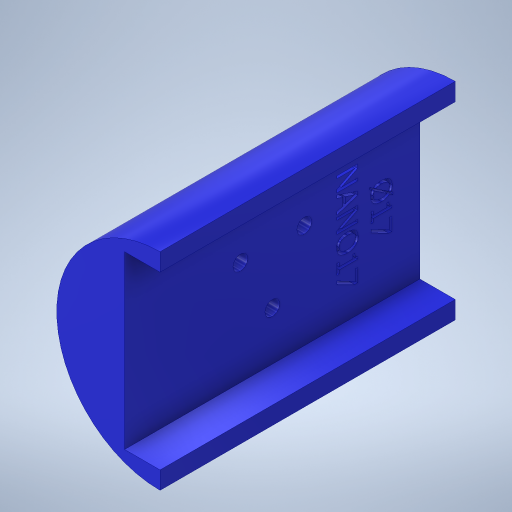
# Autodesk Inventor part: NANO17Shell18_B
Saved by Autodesk Inventor 2023 (Build 270158000, 158)
## iProperties
Created: 2016-07-01
Part Number: NANO17Shell18_B
Material: ABS Plastic
Document SubType Name: Modeling
Designer: Administrateur
Density: 1.06 g/cm^3
Appearance: Blue - Wall Paint - Glossy
Author: Administrateur
Autodesk Inventor part; units mm, degrees
ref_plane "XZ Plane" through (0, 0, 0) normal (0, 1, 0) x (-1, 0, 0)
sketch "Sketch1" plane through (0, 0, 0) normal (0, 0, 1) x (1, 0, 0)
  arc A0 (0, 17.5) -> (0, -17.5) centre (0, 0) ccw
  line L0 (0, 17.5) -> (0, 14.5)
  line L1 (0, 14.5) -> (-6, 14.5)
  line L2 (-6, 14.5) -> (-6, 0)
  line L3 (-46.5484, 0) -> (26.4312, 0) construction
  line L4 (0, -17.5) -> (0, -14.5)
  line L5 (0, -14.5) -> (-6, -14.5)
  line L6 (-6, -14.5) -> (-6, 0)
  dimension "d2" = 17.5
  dimension "d3" = 29
  dimension "d4" = 6
  dimension "d27" = 14.5
  dimension "d28" = 3
  constraints: 14 end point, 2 horizontal, 2 point on circle, 2 symmetric about line, 1 centre point, 1 coincident, 1 perpendicular, 1 vertical
  measures "d2" radius of A0
  measures "d3" distance between parallel lines of L5 L1
  measures "d4" distance of L0.end L1.end
  measures "d27" distance of L1.end L2.end
  measures "d28" distance of L0.start L0.end
extrude "Extrusion1" add sketch "Sketch1" along normal blind 50
sketch "Sketch2" plane through (-6, -14.5, 0) normal (1, 0, 0) x (0, 0, -1)
  line L0 (-25, 14.5) -> (-50, 14.5) construction
  line L1 (-50, 32) -> (-50, -3) construction
  line L2 (0, 32) -> (-50, 32) construction
  line L3 (-25, 32) -> (-25, -3) construction
  line L4 (0, -3) -> (-50, -3) construction
  circle A0 centre (-25, 14.5) radius 6.25 construction
  line L5 (-25, 14.5) -> (-30.4127, 17.625) construction
  line L6 (-25, 14.5) -> (-25, 8.25) construction
  line L7 (-25, 14.5) -> (-19.5873, 17.625) construction
  point P0 (0, 14.5)
  dimension "d6" = 12.5
  dimension "d7" = 30
  dimension "d10" = 360
  constraints: 10 end point, 4 coincident, 4 midpoint, 13 other
  measures "d7" angle of L0 L5
hole "Hole1" at (-6, -6.25, 25) at (-6, 3.125, 19.5873) at (-6, 3.125, 30.4127) direction (-1, 0, 0) diameter 2.5 end through all
ref_plane "Work Plane1" through (-17.5, 0, 0) normal (1, 0, 0) x (0, 1, 0)
sketch "Sketch3" plane through (-17.5, 0, 0) normal (1, 0, 0) x (0, 1, 0)
  line L0 (17.5, 0) -> (-17.5, 0) projected
  line L1 (-17.5, 0) -> (-17.5, 50) projected
  line L2 (17.5, 50) -> (-17.5, 50) projected
  line L3 (17.5, 0) -> (17.5, 50) projected
  circle A0 centre (3.125, 30.4127) radius 1.25 projected
  circle A1 centre (3.125, 19.5873) radius 1.25 projected
  line L4 (3.125, 30.4127) -> (3.125, 19.5873) construction
  circle A2 centre (-6.25, 25) radius 1.25 projected
  line L5 (3.125, 19.5873) -> (-6.25, 25) construction
  line L6 (-6.25, 25) -> (3.125, 30.4127) construction
  point P0 (0, 0)
  point P1 (3.125, 30.4127)
  point P2 (3.125, 19.5873)
  point P3 (-6.25, 25)
  constraints: 6 end point, 3 coincident, 3 horizontal alignment, 3 other
ref_plane "Work Plane2" through (-10, 0, 0) normal (1, 0, 0) x (0, 1, 0)
hole "Hole2" at (-17.5, 3.125, 30.4127) at (-17.5, 3.125, 19.5873) at (-17.5, -6.25, 25) direction (1, 0, 0) diameter 5 depth 7.5
sketch "Esquisse4" plane through (-6, -14.5, 0) normal (1, 0, 0) x (0, 0, -1)
  line L0 (-4.5555, 21.4204) -> (-4.5555, 5.6534) construction
  line L1 (-4.5555, 5.6534) -> (-13.9713, 5.6534) construction
  line L2 (-13.9713, 5.6534) -> (-13.9713, 21.4204) construction
  line L3 (-13.9713, 21.4204) -> (-4.5555, 21.4204) construction
  spline S0 degree 2 poles (-6.521, 14.6161) (-7.3889, 14.6161) (-8.3448, 15.4613) (-8.3448, 16.1647) knots 0 0 0 1 2 2 2
  spline S1 degree 2 poles (-8.3448, 16.1647) (-8.3448, 16.4228) (-8.2086, 16.8681) (-8.0838, 17.0468) knots 0 0 0 1 2 2 2
  line L4 (-8.0838, 17.0468) -> (-8.5433, 17.3588)
  line L5 (-8.5433, 17.3588) -> (-8.5433, 17.7049)
  line L6 (-8.5433, 17.7049) -> (-7.8909, 17.2624)
  spline S2 degree 2 poles (-7.8909, 17.2624) (-7.6584, 17.4723) (-6.972, 17.7105) (-6.521, 17.7105) knots 0 0 0 1 2 2 2
  spline S3 degree 2 poles (-6.521, 17.7105) (-5.6559, 17.7105) (-4.6973, 16.8625) (-4.6973, 16.1647) knots 0 0 0 1 2 2 2
  spline S4 degree 2 poles (-4.6973, 16.1647) (-4.6973, 15.8953) (-4.8277, 15.4755) (-4.9554, 15.2883) knots 0 0 0 1 2 2 2
  line L7 (-4.9554, 15.2883) -> (-4.5555, 15.0189)
  line L8 (-4.5555, 15.0189) -> (-4.5555, 14.67)
  line L9 (-4.5555, 14.67) -> (-5.1454, 15.0728)
  spline S5 degree 2 poles (-5.1454, 15.0728) (-5.378, 14.8572) (-6.053, 14.6161) (-6.521, 14.6161) knots 0 0 0 1 2 2 2
  spline S6 degree 2 poles (-6.521, 15.0955) (-6.1977, 15.0955) (-5.69, 15.2259) (-5.5226, 15.3337) knots 0 0 0 1 2 2 2
  line L10 (-5.5226, 15.3337) -> (-7.7264, 16.8086)
  spline S7 degree 2 poles (-7.7264, 16.8086) (-7.8342, 16.6753) (-7.942, 16.3746) (-7.942, 16.1619) knots 0 0 0 1 2 2 2
  spline S8 degree 2 poles (-7.942, 16.1619) (-7.942, 15.6769) (-7.2102, 15.0955) (-6.521, 15.0955) knots 0 0 0 1 2 2 2
  spline S9 degree 2 poles (-5.3099, 15.5266) (-5.205, 15.6485) (-5.1, 15.969) (-5.1, 16.1619) knots 0 0 0 1 2 2 2
  spline S10 degree 2 poles (-5.1, 16.1619) (-5.1, 16.6498) (-5.8233, 17.2312) (-6.521, 17.2312) knots 0 0 0 1 2 2 2
  spline S11 degree 2 poles (-6.521, 17.2312) (-6.8387, 17.2312) (-7.3322, 17.1092) (-7.508, 16.9986) knots 0 0 0 1 2 2 2
  line L11 (-7.508, 16.9986) -> (-5.3099, 15.5266)
  line L12 (-8.271, 12.2223) -> (-8.271, 13.9297)
  line L13 (-8.271, 13.9297) -> (-7.9136, 13.9297)
  line L14 (-7.9136, 13.9297) -> (-7.9136, 13.2944)
  line L15 (-7.9136, 13.2944) -> (-5.568, 13.2944)
  line L16 (-5.568, 13.2944) -> (-5.568, 13.9297)
  line L17 (-5.568, 13.9297) -> (-5.2475, 13.9297)
  spline S12 degree 2 poles (-5.2475, 13.9297) (-5.2475, 13.5695) (-5.0433, 13.2292) (-4.7597, 13.2065) knots 0 0 0 1 2 2 2
  line L18 (-4.7597, 13.2065) -> (-4.7597, 12.8434)
  line L19 (-4.7597, 12.8434) -> (-7.9136, 12.8434)
  line L20 (-7.9136, 12.8434) -> (-7.9136, 12.2223)
  line L21 (-7.9136, 12.2223) -> (-8.271, 12.2223)
  line L22 (-5.2957, 9.3803) -> (-8.271, 10.8949)
  line L23 (-8.271, 10.8949) -> (-8.271, 11.3941)
  line L24 (-8.271, 11.3941) -> (-5.1823, 9.7944)
  line L25 (-5.1823, 9.7944) -> (-5.1823, 11.6011)
  line L26 (-5.1823, 11.6011) -> (-4.771, 11.6011)
  line L27 (-4.771, 11.6011) -> (-4.771, 9.3803)
  line L28 (-4.771, 9.3803) -> (-5.2957, 9.3803)
  line L29 (-14.0337, 19.6647) -> (-14.0337, 20.1866)
  line L30 (-14.0337, 20.1866) -> (-11.0158, 21.7352)
  line L31 (-11.0158, 21.7352) -> (-14.0337, 21.7352)
  line L32 (-14.0337, 21.7352) -> (-14.0337, 22.1692)
  line L33 (-14.0337, 22.1692) -> (-10.5337, 22.1692)
  line L34 (-10.5337, 22.1692) -> (-10.5337, 21.5083)
  line L35 (-10.5337, 21.5083) -> (-13.3047, 20.0987)
  line L36 (-13.3047, 20.0987) -> (-10.5337, 20.0987)
  line L37 (-10.5337, 20.0987) -> (-10.5337, 19.6647)
  line L38 (-10.5337, 19.6647) -> (-14.0337, 19.6647)
  line L39 (-14.0337, 19.3329) -> (-10.5337, 18.153)
  line L40 (-10.5337, 18.153) -> (-10.5337, 17.5801)
  line L41 (-10.5337, 17.5801) -> (-14.0337, 16.4002)
  line L42 (-14.0337, 16.4002) -> (-14.0337, 16.8908)
  line L43 (-14.0337, 16.8908) -> (-13.0551, 17.2085)
  line L44 (-13.0551, 17.2085) -> (-13.0551, 18.5444)
  line L45 (-13.0551, 18.5444) -> (-14.0337, 18.8621)
  line L46 (-14.0337, 18.8621) -> (-14.0337, 19.3329)
  line L47 (-12.6581, 17.3361) -> (-11.0102, 17.8779)
  line L48 (-11.0102, 17.8779) -> (-12.6581, 18.4168)
  line L49 (-12.6581, 18.4168) -> (-12.6581, 17.3361)
  line L50 (-14.0337, 13.5639) -> (-14.0337, 14.0857)
  line L51 (-14.0337, 14.0857) -> (-11.0158, 15.6344)
  line L52 (-11.0158, 15.6344) -> (-14.0337, 15.6344)
  line L53 (-14.0337, 15.6344) -> (-14.0337, 16.0683)
  line L54 (-14.0337, 16.0683) -> (-10.5337, 16.0683)
  line L55 (-10.5337, 16.0683) -> (-10.5337, 15.4075)
  line L56 (-10.5337, 15.4075) -> (-13.3047, 13.9978)
  line L57 (-13.3047, 13.9978) -> (-10.5337, 13.9978)
  line L58 (-10.5337, 13.9978) -> (-10.5337, 13.5639)
  line L59 (-10.5337, 13.5639) -> (-14.0337, 13.5639)
  spline S13 degree 2 poles (-10.9336, 10.3787) (-11.1662, 10.1801) (-11.8469, 9.9589) (-12.2837, 9.9589) knots 0 0 0 1 2 2 2
  spline S14 degree 2 poles (-12.2837, 9.9589) (-12.7091, 9.9589) (-13.3983, 10.1745) (-13.6309, 10.3787) knots 0 0 0 1 2 2 2
  spline S15 degree 2 poles (-13.6309, 10.3787) (-13.8748, 10.5942) (-14.1074, 11.1643) (-14.1074, 11.5075) knots 0 0 0 1 2 2 2
  spline S16 degree 2 poles (-14.1074, 11.5075) (-14.1074, 11.8621) (-13.8663, 12.4293) (-13.6309, 12.6364) knots 0 0 0 1 2 2 2
  spline S17 degree 2 poles (-13.6309, 12.6364) (-13.3983, 12.8378) (-12.7148, 13.0533) (-12.2837, 13.0533) knots 0 0 0 1 2 2 2
  spline S18 degree 2 poles (-12.2837, 13.0533) (-11.844, 13.0533) (-11.1747, 12.8349) (-10.9336, 12.6335) knots 0 0 0 1 2 2 2
  spline S19 degree 2 poles (-10.9336, 12.6335) (-10.701, 12.4293) (-10.4599, 11.8592) (-10.4599, 11.5075) knots 0 0 0 1 2 2 2
  spline S20 degree 2 poles (-10.4599, 11.5075) (-10.4599, 11.1502) (-10.7095, 10.5772) (-10.9336, 10.3787) knots 0 0 0 1 2 2 2
  spline S21 degree 2 poles (-12.2837, 10.4439) (-11.9376, 10.4439) (-11.4016, 10.5942) (-11.2257, 10.7304) knots 0 0 0 1 2 2 2
  spline S22 degree 2 poles (-11.2257, 10.7304) (-11.0442, 10.8694) (-10.8627, 11.2608) (-10.8627, 11.5047) knots 0 0 0 1 2 2 2
  spline S23 degree 2 poles (-10.8627, 11.5047) (-10.8627, 11.7571) (-11.0385, 12.1372) (-11.2257, 12.2818) knots 0 0 0 1 2 2 2
  spline S24 degree 2 poles (-11.2257, 12.2818) (-11.4044, 12.4208) (-11.9433, 12.5683) (-12.2837, 12.5683) knots 0 0 0 1 2 2 2
  spline S25 degree 2 poles (-12.2837, 12.5683) (-12.9729, 12.5683) (-13.7047, 11.9897) (-13.7047, 11.5047) knots 0 0 0 1 2 2 2
  spline S26 degree 2 poles (-13.7047, 11.5047) (-13.7047, 11.0197) (-12.9729, 10.4439) (-12.2837, 10.4439) knots 0 0 0 1 2 2 2
  line L60 (-14.0337, 7.5651) -> (-14.0337, 9.2725)
  line L61 (-14.0337, 9.2725) -> (-13.6763, 9.2725)
  line L62 (-13.6763, 9.2725) -> (-13.6763, 8.6372)
  line L63 (-13.6763, 8.6372) -> (-11.3307, 8.6372)
  line L64 (-11.3307, 8.6372) -> (-11.3307, 9.2725)
  line L65 (-11.3307, 9.2725) -> (-11.0102, 9.2725)
  spline S27 degree 2 poles (-11.0102, 9.2725) (-11.0102, 8.9123) (-10.806, 8.572) (-10.5223, 8.5493) knots 0 0 0 1 2 2 2
  line L66 (-10.5223, 8.5493) -> (-10.5223, 8.1862)
  line L67 (-10.5223, 8.1862) -> (-13.6763, 8.1862)
  line L68 (-13.6763, 8.1862) -> (-13.6763, 7.5651)
  line L69 (-13.6763, 7.5651) -> (-14.0337, 7.5651)
  line L70 (-11.0584, 4.7231) -> (-14.0337, 6.2377)
  line L71 (-14.0337, 6.2377) -> (-14.0337, 6.7369)
  line L72 (-14.0337, 6.7369) -> (-10.9449, 5.1372)
  line L73 (-10.9449, 5.1372) -> (-10.9449, 6.9439)
  line L74 (-10.9449, 6.9439) -> (-10.5337, 6.9439)
  line L75 (-10.5337, 6.9439) -> (-10.5337, 4.7231)
  line L76 (-10.5337, 4.7231) -> (-11.0584, 4.7231)
  point P0 (0, 14.5)
  constraints: 2 other
extrude "Extrusion2" cut sketch "Esquisse4" against normal blind 1
equation "\"d27\" = 0.5 * d3"
equation "\"d28\" = -0.5 * d3 + d2"
body "Solid1"
